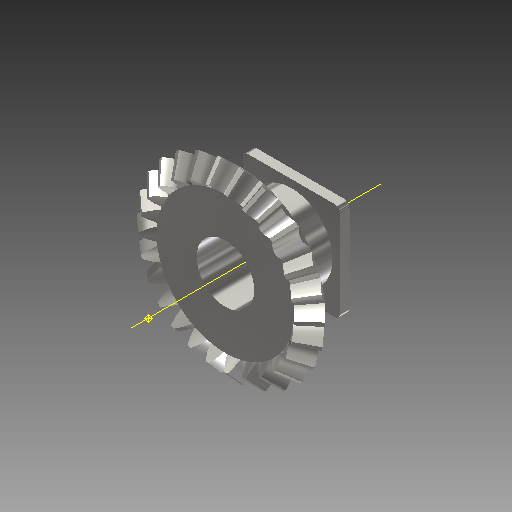
# Autodesk Inventor part: Kegelrad1
Saved by Autodesk Inventor 2018 (Build 220112000, 112)
## iProperties
Created: 2017-04-26
Part Number: Kegelrad1
Material: Siliziumnitrid
Document SubType Name: Modeling
Designer: Jochen Alt
Categories: <?xml version="1.0" encoding="UTF-16"?> <MemberInstance><Categories><FamilyTemplate><FamilyTemplateParameter ValueType="xs:double" Id="1" ObjectReferenceKey="da_z" ObjectType="kUserParameterObject"/><FamilyTemplateParameter ValueType="xs:double" Id="2" ObjectReferenceKey="da_b" ObjectType="kUserParameterObject"/><FamilyTemplateParameter ValueType="xs:double" Id="3" ObjectReferenceKey="da_beta" ObjectType="kUserParameterObject"/><FamilyTemplateParameter ValueType="xs:double" Id="4" ObjectReferenceKey="da_dae" ObjectType="kUserParameterObject"/><FamilyTemplateParameter ValueType="xs:double" Id="5" ObjectReferenceKey="da_ve" ObjectType="kUserParameterObject"/><FamilyTemplateParameter ValueType="xs:double" Id="6" ObjectReferenceKey="da_omega" ObjectType="kUserParameterObject"/><FamilyTemplateParameter ValueType="xs:string" Id="7" ObjectReferenceKey="EAIAABAAAAAAHwAAAAAAAIAAAAAAAAAA" ObjectType="83914240" SubObjectId="SurfaceGeometry"/></FamilyTemplate><ParamToTemplateMap><ParamToTemplate CategoryParameter="//CategoryParameter[@InternalName='046C89C9-8512-4d59-83FE-43B91F4F132A']" TemplateParameter="1"/><ParamToTemplate CategoryParameter="//CategoryParameter[@InternalName='2552DF32-E462-4b46-AEBF-C6C7768E72AC']" TemplateParameter="2"/><ParamToTemplate CategoryParameter="//CategoryParameter[@InternalName='C9EE641D-15FC-4fae-A226-E94C4372FDD7']" TemplateParameter="3"/><ParamToTemplate><ParamToTemplate CategoryParameter="//CategoryParameter[@InternalName='00B6519A-459B-49c7-AD84-2E56D39A5744']" ConstantValue="0.000000"/></ParamToTemplate><ParamToTemplate><ParamToTemplate CategoryParameter="//CategoryParameter[@InternalName='04B31F0E-C7A6-4894-AA32-9629BEFACF47']" ConstantValue="1.000000"/></ParamToTemplate><ParamToTemplate><ParamToTemplate CategoryParameter="//CategoryParameter[@InternalName='43CBEC2E-7847-49e7-A936-2F7889FCB2D9']" ConstantValue="0.200000"/></ParamToTemplate><ParamToTemplate><ParamToTemplate CategoryParameter="//CategoryParameter[@InternalName='B1EFC894-105D-4ebd-86BF-FA20ED196853']" ConstantValue="0.266800"/></ParamToTemplate><ParamToTemplate><ParamToTemplate CategoryParameter="//CategoryParameter[@InternalName='51175063-3D10-4879-93E8-6246FE8B403D']" ConstantValue="2060000000.000000"/></ParamToTemplate><ParamToTemplate><ParamToTemplate CategoryParameter="//CategoryParameter[@InternalName='A3A52E27-4454-46a9-B0BD-C932399B70AF']" ConstantValue="0.300000"/></ParamToTemplate><ParamToTemplate CategoryParameter="//CategoryParameter[@InternalName='2A200944-5A8C-41ca-B96E-8520D2E510F1']" TemplateParameter="4"/><ParamToTemplate><ParamToTemplate CategoryParameter="//CategoryParameter[@InternalName='1A637F62-92C8-44bc-B81F-10802510B579']" ConstantValue="2.815865"/></ParamToTemplate><ParamToTemplate CategoryParameter="//CategoryParameter[@InternalName='B52DD4BE-6863-48fb-BF58-89EF6F9EC65C']" TemplateParameter="5"/><ParamToTemplate><ParamToTemplate CategoryParameter="//CategoryParameter[@InternalName='3956BFF2-84D2-457d-93C2-9B0613DEBA67']" ConstantValue="1.211140"/></ParamToTemplate><ParamToTemplate CategoryParameter="//CategoryParameter[@InternalName='739CFA02-461B-4bf8-8049-181FCAD8B28F']" TemplateParameter="6"/><ParamToTemplate><ParamToTemplate CategoryParameter="//CategoryParameter[@InternalName='A27E999F-E2CE-4481-8A2A-EBF499C4C3C5']" ConstantValue="0.000000"/></ParamToTemplate><ParamToTemplate><ParamToTemplate CategoryParameter="//CategoryParameter[@InternalName='9E1B4470-B2D3-4ff1-B813-535BB4CDF51A']" ConstantValue="3520000.000000"/></ParamToTemplate><ParamToTemplate><ParamToTemplate CategoryParameter="//CategoryParameter[@InternalName='F8452263-BFF6-458c-9FB1-07C4B99E95CD']" ConstantValue="11400000.000000"/></ParamToTemplate><ParamToTemplate><ParamToTemplate CategoryParameter="//CategoryParameter[@InternalName='3E3BB259-FD49-497f-8171-6EBC954A3479']" ConstantValue="2.000000"/></ParamToTemplate><ParamToTemplate CategoryParameter="//CategoryParameter[@InternalName='27C3BAF2-7550-4e4b-AE2C-0DB134B7D9B7']" TemplateParameter="7"/></ParamToTemplateMap><Category DisplayName="Gear" InternalName="DC85795E-93AB-48d5-8EEE-5A27447B64BD" Mnemonic="Gear"><CategoryParameter DisplayName="z" InternalName="046C89C9-8512-4d59-83FE-43B91F4F132A" Mnemonic="z"/><CategoryParameter DisplayName="b" InternalName="2552DF32-E462-4b46-AEBF-C6C7768E72AC" Mnemonic="b"/><CategoryParameter DisplayName="||b|" InternalName="C9EE641D-15FC-4fae-A226-E94C4372FDD7" Mnemonic="beta"/><CategoryParameter DisplayName="x" InternalName="00B6519A-459B-49c7-AD84-2E56D39A5744" Mnemonic="x"/><CategoryParameter DisplayName="a*" InternalName="04B31F0E-C7A6-4894-AA32-9629BEFACF47" Mnemonic="a"/><CategoryParameter DisplayName="c*" InternalName="43CBEC2E-7847-49e7-A936-2F7889FCB2D9" Mnemonic="c"/><CategoryParameter DisplayName="r|.f|*" InternalName="B1EFC894-105D-4ebd-86BF-FA20ED196853" Mnemonic="rf"/><CategoryParameter DisplayName="E" InternalName="51175063-3D10-4879-93E8-6246FE8B403D" Mnemonic="E"/><CategoryParameter DisplayName="||m|" InternalName="A3A52E27-4454-46a9-B0BD-C932399B70AF" Mnemonic="mi"/><Category DisplayName="BevelGear" InternalName="0C98F69A-0C2B-4791-B2FE-7691BB227E77" Mnemonic="BevelGear"><CategoryParameter DisplayName="d|.ae|" InternalName="2A200944-5A8C-41ca-B96E-8520D2E510F1" Mnemonic="dae"/><CategoryParameter DisplayName="d|.ai|" InternalName="1A637F62-92C8-44bc-B81F-10802510B579" Mnemonic="dai"/><CategoryParameter DisplayName="A|.e|" InternalName="B52DD4BE-6863-48fb-BF58-89EF6F9EC65C" Mnemonic="ve"/><CategoryParameter DisplayName="A|.i|" InternalName="3956BFF2-84D2-457d-93C2-9B0613DEBA67" Mnemonic="vi"/><CategoryParameter DisplayName="||S|" InternalName="739CFA02-461B-4bf8-8049-181FCAD8B28F" Mnemonic="omega"/><CategoryParameter DisplayName="x|.t|" InternalName="A27E999F-E2CE-4481-8A2A-EBF499C4C3C5" Mnemonic="xt"/><CategoryParameter DisplayName="||s||.Flim|" InternalName="9E1B4470-B2D3-4ff1-B813-535BB4CDF51A" Mnemonic="sFlim"/><CategoryParameter DisplayName="||s||.Hlim|" InternalName="F8452263-BFF6-458c-9FB1-07C4B99E95CD" Mnemonic="sHlim"/><CategoryParameter DisplayName="Typ" InternalName="3E3BB259-FD49-497f-8171-6EBC954A3479" Mnemonic="type"/><CategoryParameter DisplayName="PitchDiameter" InternalName="27C3BAF2-7550-4e4b-AE2C-0DB134B7D9B7" Mnemonic="IDS_PITCHDIAM"/></Category></Category></Categories></MemberInstance>
Mass: 14.0084 g
Surface Area: 31.2587 cm^2
Volume: 4.40514 cm^3
Density: 3.18 g/cm^3
Appearance: Titan
CustomPartVersion: 1
Author: Jochen Alt
Autodesk Inventor part; units mm, degrees
ref_plane "Netzebene2" through (0, 0, 0) normal (0.9927089, 0.1205367, 0) x (0, 0, 1)
sketch "Skizze des Zahnradkörpers" plane through (0, 0, 0) normal (1, 0, 0) x (0, 1, 0)
  line L0 (0, 0) -> (15.2103, -16.7062) construction
  line L1 (15.2103, -16.7062) -> (17.1164, -14.724)
  line L2 (17.1164, -14.724) -> (0, 0) construction
  line L3 (16.25, -15.625) -> (0, 0) construction
  line L4 (12.5115, -13.742) -> (14.0793, -12.1114)
  line L5 (15.2103, -16.7062) -> (12.5115, -13.742)
  line L6 (17.1164, -14.724) -> (14.0793, -12.1114)
  line L7 (0, -20.0475) -> (0, 3.3412) projected
  line L8 (0, -15.625) -> (17.1164, -15.625) construction
  dimension "d0" = 32.5
  dimension "d1" = 30.4207
  dimension "d2" = 34.2328
  dimension "d3" = 4
  dimension "d4" = 14.724
  constraints: 16 end point, 4 point on line, 3 perpendicular, 2 collinear, 1 horizontal alignment, 1 vertical alignment
  measures "d0" diameter of L3.start L7
  measures "d1" diameter of L0.end L7
  measures "d2" diameter of L1.end L7
  measures "d3" distance between parallel lines of L1 L4
  measures "d4" vertical distance of L1.end L0.start
revolve "Zahnradkörper" add sketch "Skizze des Zahnradkörpers" angle 360 about axis through (0, 0, 0) along (0, 0, 1)
ref_plane "Zahnebene" through (0, 16.25, -15.625) normal (0, -0.7208331, 0.6931087) x (1, 0, 0)
sketch "Startskizze" plane through (0, 16.25, -15.625) normal (0, -0.7208331, 0.6931087) x (1, 0, 0)
  line L0 (0, -28.5497) -> (0, 7.1824) projected
  arc A0 (-0.2795, -1.83) -> (-2.3169, 1.9696) centre (-10.1369, -4.6695) ccw
  arc A1 (2.3169, 1.9696) -> (0.2795, -1.83) centre (10.1369, -4.6695) ccw
  line L1 (-0.2795, -1.83) -> (0.2795, -1.83)
  arc A2 (2.3169, 1.9696) -> (-2.3169, 1.9696) centre (0, -23.4451) ccw
  dimension "d7" = 10.2582
  dimension "d8" = 10.1369
  dimension "d9" = 18.7756
  dimension "d57" = 25.5201
  dimension "d58" = 21.6151
  constraints: 6 point on circle, 3 centre point, 3 symmetric about line, 2 end point, 1 coincident, 1 perpendicular, 1 other
  measures "d7" radius of A0
  measures "d8" horizontal distance of point (0, -23.445) A0.centre
  measures "d9" vertical distance of point (0, -23.445) A0.centre
  measures "d57" radius of A2
  measures "d58" distance from line of A2.centre L1
ref_plane "Endebene" through (0, 13.2676, -12.7573) normal (0, -0.7208331, 0.6931087) x (1, 0, 0)
sketch "Endskizze" plane through (0, 13.2676, -12.7573) normal (0, -0.7208331, 0.6931087) x (1, 0, 0)
  line L0 (0, -22.0485) -> (0, 5.5762) projected
  arc A0 (-0.2285, -1.4725) -> (-1.8939, 1.6335) centre (-8.2865, -3.7937) ccw
  arc A1 (1.8939, 1.6335) -> (0.2285, -1.4725) centre (8.2865, -3.7937) ccw
  line L1 (-0.2285, -1.4725) -> (0.2285, -1.4725)
  arc A2 (1.8939, 1.6335) -> (-1.8939, 1.6335) centre (0, -19.1421) ccw
  dimension "d12" = 8.3857
  dimension "d15" = 8.2866
  dimension "d16" = 15.3484
  dimension "d59" = 20.8618
  dimension "d60" = 17.6696
  constraints: 6 point on circle, 3 centre point, 3 symmetric about line, 2 end point, 1 coincident, 1 other
  measures "d12" radius of A0
  measures "d15" horizontal distance of A0.centre point (0, -19.142)
  measures "d16" vertical distance of A0.centre point (0, -19.142)
  measures "d59" radius of A2
  measures "d60" distance from line of A2.centre L1
loft "Loft" cut profiles "Startskizze", "Endskizze"
pattern_circular "Circular Pattern" count 26 over 360 about axis through (0, 0, 0) along (0, 0, 1) of "Loft"
sketch3d "3D-Skizze rechts"
ref_plane "Endebene rechts" through (-1.4139, 13.192, -12.7573) normal (0.0768159, -0.7167284, 0.6931087) x (0.9943057, 0.1065655, 0)
sketch "Endskizze rechts" plane through (-1.4139, 13.192, -12.7573) normal (0.0768159, -0.7167284, 0.6931087) x (0.9943057, 0.1065655, 0)
  arc A0 (-0.2285, -1.4725) -> (-1.8939, 1.6335) centre (-8.2865, -3.7937) ccw
  line L0 (0, -24.908) -> (0, 7.3958) projected
  arc A1 (1.8939, 1.6335) -> (0.2285, -1.4725) centre (8.2865, -3.7937) ccw
  line L1 (-0.2285, -1.4725) -> (0.2285, -1.4725)
  arc A2 (1.8939, 1.6335) -> (-1.8939, 1.6335) centre (0, -19.1421) ccw
  dimension "d70" = 8.2866
  dimension "d71" = 15.3484
  dimension "d72" = 8.3857
  dimension "d73" = 17.6696
  dimension "d74" = 20.8618
  constraints: 6 point on circle, 3 centre point, 3 symmetric about line, 2 end point, 1 coincident, 1 perpendicular, 1 other
  measures "d70" horizontal distance of A2.centre A0.centre
  measures "d71" vertical distance of point (0, -19.142) A0.centre
  measures "d72" radius of A0
  measures "d73" distance from line of point (0, -19.142) L1
  measures "d74" radius of A2
feature "Erhebung rechts" [suppressed]
pattern_circular "Runde Anordnung rechts" [suppressed]
sketch3d "3D-Skizze links"
ref_plane "Endebene links" through (1.4372, 13.192, -12.7689) normal (-0.0780422, -0.7163444, 0.6933687) x (0.9941178, -0.1083042, 0)
sketch "Endskizze links" plane through (1.4372, 13.192, -12.7689) normal (-0.0780422, -0.7163444, 0.6933687) x (0.9941178, -0.1083042, 0)
  line L0 (0, -26.074) -> (0, 8.5744) projected
  arc A0 (-0.2285, -1.4659) -> (-1.8939, 1.6402) centre (-8.2865, -3.7871) ccw
  arc A1 (1.8939, 1.6402) -> (0.2285, -1.4659) centre (8.2865, -3.7871) ccw
  line L1 (-0.2285, -1.4659) -> (0.2285, -1.4659)
  ellipse E0 centre (0, -8.7273) end of major axis (14.0793, -8.7273) minor radius 9.7622 projected
  arc A2 (1.8939, 1.6402) -> (-1.8939, 1.6402) centre (0, -19.1355) ccw
  dimension "d56" = 9.7622
  dimension "d30" = 8.3857
  dimension "d31" = 8.2866
  dimension "d32" = 15.3484
  dimension "d61" = 20.8618
  dimension "d62" = 17.6696
  constraints: 6 point on circle, 3 centre point, 3 symmetric about line, 2 end point, 1 coincident, 2 other
  measures "d30" radius of A0
  measures "d31" horizontal distance of point (0, -19.135) A0.centre
  measures "d32" vertical distance of A0.centre point (0, -19.135)
  measures "d61" radius of A2
  measures "d62" distance from line of point (0, -19.135) L1
feature "Erhebung links" [suppressed]
pattern_circular "Runde Anordnung links" [suppressed]
sketch "Körperskizze" plane through (0, 0, 0) normal (1, 0, 0) x (0, 1, 0)
  line L0 (0, -17.4473) -> (0, -12.2598) projected
  line L1 (15.2103, -16.7062) -> (12.5115, -13.742) projected
  line L2 (12.5115, -13.742) -> (0, -13.742)
  line L3 (15.2103, -16.7062) -> (0, -16.7062)
  constraints: 4 end point, 2 perpendicular, 2 point on line
revolve "Festkörper" add sketch "Körperskizze" angle 360 about axis through (0, 0, 0) along (0, 0, 1)
sketch "Sketch6" plane through (0, 0, 0) normal (1, 0, 0) x (0, 1, 0)
  line L0 (16.25, -15.625) -> (0, 0) projected
  line L1 (0, -18.75) -> (0, 3.125) projected
surface revolve "Flankendurchmesser" sketch "Sketch6" angle 360 about axis through (0, 0, 0) along (0, 0, 1) shown no curves L0
sketch "Skizze8" plane through (0, 0, -16.7062) normal (0, 0, -1) x (-1, 0, 0)
  arc A0 (3.2706, 14.8546) -> (0.3794, 15.2056) centre (0, 0) ccw projected
  circle A1 centre (0, 0) radius 7.5
  dimension "d94" = 15
  constraints: 1 centre point, 1 coincident
  measures "d94" diameter of A1
extrude "Extrusion1" add sketch "Skizze8" along normal blind 9.05
sketch "Skizze9" plane through (0, 0, -25.7562) normal (0, 0, -1) x (-1, 0, 0)
  circle A0 centre (0, 0) radius 7.5 projected
  line L0 (8.9, -8.9) -> (-8.9, -8.9)
  line L1 (-8.9, -8.9) -> (-8.9, 8.9)
  line L2 (-8.9, 8.9) -> (8.9, 8.9)
  line L3 (8.9, 8.9) -> (8.9, -8.9)
  line L4 (8.9, -8.9) -> (-8.9, 8.9) construction
  line L5 (-8.9, -8.9) -> (8.9, 8.9) construction
  dimension "d97" = 17.8
  dimension "d98" = 17.8
  constraints: 12 end point, 2 midpoint, 2 parallel, 1 horizontal, 1 perpendicular
  measures "d97" distance of L1.end L2.end
  measures "d98" distance of L0.end L1.end
extrude "Extrusion2" add sketch "Skizze9" along normal blind 1.7 contours A0 | L0 L1 L2 L3
fillet "Rundung1" radius 1 4 edges at (8.9, 8.9, -26.6062) (8.9, -8.9, -26.6062) (-8.9, -8.9, -26.6062) (-8.9, 8.9, -26.6062)
chamfer "Fase1" distance 7.7 distance2 5 1 edges at (7.5, 0, -16.7062) measured on face at (-9.9654, -1.1676, -16.7062)
sketch "Skizze10" plane through (0, 0, -13.742) normal (0, 0, 1) x (1, 0, 0)
  arc A0 (2.6965, 12.2174) -> (0.3056, 12.5077) centre (0, 0) ccw projected
  circle A1 centre (0, 0) radius 5.25
  dimension "d105" = 10.5
  constraints: 1 centre point, 1 coincident
  measures "d105" diameter of A1
extrude "Extrusion3" cut sketch "Skizze10" against normal through all
sketch "Skizze11" plane through (0, 0, -27.4562) normal (0, 0, -1) x (-1, 0, 0)
  line L0 (11.0104, -2.1054) -> (3.0104, -2.1054)
  line L1 (3.0104, -2.1054) -> (3.0104, 2.1054)
  line L2 (3.0104, 2.1054) -> (11.0104, 2.1054)
  line L3 (11.0104, 2.1054) -> (11.0104, -2.1054)
  line L4 (11.0104, -2.1054) -> (3.0104, 2.1054) construction
  line L5 (3.0104, -2.1054) -> (11.0104, 2.1054) construction
  point P0 (7.0104, 0)
  dimension "d108" = 8
  constraints: 12 end point, 2 midpoint, 2 parallel, 1 horizontal, 1 perpendicular
  measures "d108" distance of L1.end L2.end
extrude "Extrusion4" cut sketch "Skizze11" against normal up to surface (1.7 mm away)
equation "\"d0\" = da_de"
equation "\"d1\" = da_dfe"
equation "\"d2\" = da_dae"
equation "\"d3\" = da_b"
equation "\"d4\" = da_ve"
equation "\"d7\" = fd_rr"
equation "\"d8\" = fd_x"
equation "\"d9\" = fd_y"
equation "\"d57\" = 0.5 * fd_dva + 0.3 * da_he"
equation "\"d58\" = 0.5 * fd_dva - 1.12 * da_he"
equation "\"da_teethtype\" = 0"
equation "\"da_b\" = 4"
equation "\"da_de\" = 32.5"
equation "\"da_dae\" = 34.23277"
equation "\"da_dfe\" = 30.42067"
equation "\"da_le\" = 22.54336"
equation "\"da_omega\" = 90deg"
equation "\"da_beta\" = 0"
equation "\"da_delta\" = 46.123303deg"
equation "\"da_alpha\" = 25deg"
equation "\"da_he\" = 2.75"
equation "\"da_ve\" = 14.72396"
equation "\"da_zv\" = 37.512153"
equation "\"fd_loft\" = da_b + 0.05 * da_he"
equation "\"fd_x\" = fd_x1 + fd_x2"
equation "\"fd_y\" = fd_y1 - fd_y2"
equation "\"fd_dd\" = fd_dva - 0.8 * da_he"
equation "\"da_dvw\" = 46.89019"
equation "\"d11\" = fd_loft"
equation "\"da_dm\" = 29.61667"
equation "\"da_x\" = 0"
equation "\"da_m\" = 1.25"
equation "\"d50\" = da_omega"
equation "\"fd_rr\" = 10.258213"
equation "\"fd_dva\" = 49.390191"
equation "\"fd_x1\" = 0.992359"
equation "\"fd_x2\" = 9.144526"
equation "\"fd_y1\" = 23.424084"
equation "\"fd_y2\" = 4.648504"
body "Solid1"
body "Srf1"
